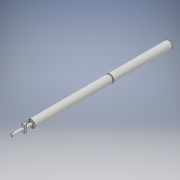
# Autodesk Inventor part: Lever
Saved by Autodesk Inventor 2018 (Build 220112000, 112)
## iProperties
Created: 2019-06-06
Part Number: Lever
Material: Generic
Document SubType Name: Modeling
Designer: aal_9
Density: 1 g/cm^3
Appearance: Default
Mass: 30.5385 g
Surface Area: 111.723 cm^2
Volume: 30.5385 cm^3
Author: aal_9
Autodesk Inventor part; units mm, degrees
ref_plane "YZ Plane" through (0, 0, 0) normal (1, 0, 0) x (0, 1, 0)
ref_plane "XZ Plane" through (0, 0, 0) normal (0, 1, 0) x (-1, 0, 0)
sketch "Sketch1" plane through (0, 0, 0) normal (0, 1, 0) x (-1, 0, 0)
  circle A0 centre (0, 0) radius 6
  dimension "d0" = 12
  constraints: 1 centre point, 1 coincident
  measures "d0" diameter of A0
extrude "Extrusion1" add sketch "Sketch1" along normal blind 250
sketch "Sketch2" plane through (0, 0, 0) normal (0, 0, 1) x (1, 0, 0)
  line L0 (-6, 0) -> (-6, 250) projected
  line L1 (-6, 155.5) -> (-4.875, 155.5)
  line L2 (-4.875, 155.5) -> (-4.875, 157)
  line L3 (-4.875, 157) -> (-6, 157)
  line L4 (-6, 157) -> (-6, 155.5)
  line L5 (0, 0) -> (0, 268.3776) construction
  line L6 (-6, 0) -> (6, 0) projected
  line L7 (6, 250) -> (-6, 250) projected
  dimension "d3" = 1.125
  dimension "d4" = 1.5
  dimension "d21" = 93
  constraints: 10 end point, 2 parallel, 1 horizontal, 1 perpendicular, 1 point on line, 1 vertical
  measures "d3" distance of L1.start L1.end
  measures "d4" distance of L1.end L2.end
  measures "d21" distance between parallel lines of L7 L3
revolve "Revolution1" cut sketch "Sketch2" angle 360 about axis through (0, 0, 0) along (0, 1, 0)
sketch "Sketch3" plane through (0, 0, 0) normal (0, 0, 1) x (1, 0, 0)
  circle A0 centre (0, 245) radius 2.5
  line L0 (6, 250) -> (-6, 250) projected
  point P0 (0, 0)
  dimension "d7" = 5
  dimension "d9" = 5
  constraints: 1 centre point
  measures "d7" diameter of A0
  measures "d9" distance from line of A0.centre L0
extrude "Extrusion2" cut sketch "Sketch3" along normal blind 2 and the other way blind 10
sketch "Sketch4" plane through (0, 250, 0) normal (0, 1, 0) x (1, 0, 0)
  point P0 (0, 0)
  point P1 (0, 0)
  constraints: 1 coincident
hole "Hole1" at (0, 250, 0) direction (0, -1, 0) diameter 2.459 depth 6 tip angle 118 thread size "M3x0.5" class "6H" standard "ANSI Metric M Profile"
sketch "Sketch5" plane through (0, 0, 0) normal (1, 0, 0) x (0, 1, 0)
  line L0 (250, -6) -> (250, 6) projected
  point P0 (0, 0)
  point P1 (220, 0)
  dimension "d22" = 30
  measures "d22" distance from line of L0 point (220, 0)
hole "Hole2" at (0, 220, 0) direction (-1, 0, 0) diameter 5 end through all
sketch "Sketch6" plane through (0, 0, 0) normal (0, -1, 0) x (1, 0, 0)
  circle A0 centre (0, 0) radius 2
  circle A1 centre (0, 0) radius 6
  dimension "d30" = 4
  dimension "d31" = 12
  constraints: 2 centre point, 2 coincident
  measures "d30" diameter of A0
  measures "d31" diameter of A1
extrude "Extrusion3" cut sketch "Sketch6" against normal blind 18.4
ref_plane "Work Plane1" through (0, 31.8, 0) normal (0, -1, 0) x (1, 0, 0)
sketch "Sketch7" plane through (0, 31.8, 0) normal (0, -1, 0) x (1, 0, 0)
  circle A0 centre (0, 0) radius 6
  circle A1 centre (0, 0) radius 2
  dimension "d35" = 12
  dimension "d36" = 4
  constraints: 2 centre point, 2 coincident
  measures "d35" diameter of A0
  measures "d36" diameter of A1
extrude "Extrusion4" cut sketch "Sketch7" along normal blind 9.4
sketch "Sketch9" plane through (0, 0, 0) normal (0, 0, 1) x (1, 0, 0)
  line L0 (2, 31.8) -> (2, 22.4) projected
  line L1 (6, 18.4) -> (-6, 18.4) projected
  line L2 (2, 22.4) -> (6, 22.4)
  line L3 (6, 22.4) -> (6, 18.4)
  line L4 (6, 18.4) -> (2, 18.4)
  line L5 (2, 18.4) -> (2, 22.4)
  line L6 (-2, 31.8) -> (-2, 22.4) projected
  line L7 (-6, 18.4) -> (-2, 18.4)
  line L8 (-2, 18.4) -> (-2, 22.4)
  line L9 (-2, 22.4) -> (-6, 22.4)
  line L10 (-6, 22.4) -> (-6, 18.4)
  point P0 (0, 0)
  dimension "d39" = 4
  constraints: 16 end point, 4 parallel, 3 point on line, 2 horizontal, 2 perpendicular
  measures "d39" distance of L8.end L9.end
extrude "Extrusion5" cut sketch "Sketch9" along normal through all both and the other way through all
sketch "Sketch10" plane through (0, 31.8, 0) normal (0, -1, 0) x (1, 0, 0)
  arc A0 (2.0552, 1.1503) -> (2.0552, -1.1503) centre (0, 0) ccw construction
  line L0 (0, 2.5) -> (0, -2.5) projected
  line L1 (2.0552, -6.3985) -> (2.6552, -6.3985)
  line L2 (2.6552, -6.3985) -> (2.6552, -2.1237)
  arc A1 (-2.0552, -2.7086) -> (2.0552, -2.7086) centre (0, 0) ccw
  arc A2 (2.6552, -2.1237) -> (2.6552, 2.1237) centre (0, 0) ccw
  line L3 (2.0552, -2.7086) -> (2.0552, -6.3985)
  line L4 (-2.0552, 7.8347) -> (-2.6552, 7.8347)
  line L5 (-2.6552, 7.8347) -> (-2.6552, 2.1237)
  line L6 (-2.0552, 2.7086) -> (-2.0552, 7.8347)
  arc A3 (2.6552, -2.1237) -> (-2.0552, 2.7086) centre (0, 0) ccw
  arc A4 (-2.6552, 2.1237) -> (2.0552, -2.7086) centre (0, 0) ccw
  arc A5 (2.0552, 2.7086) -> (-2.0552, 2.7086) centre (0, 0) ccw
  arc A6 (-2.6552, 2.1237) -> (-2.6552, -2.1237) centre (0, 0) ccw
  dimension "d59" = 0
  dimension "d60" = 0.6
  dimension "d62" = 0.6
  constraints: 16 point on circle, 12 end point, 7 centre point, 2 coincident, 2 parallel
  measures "d59" distance from line of A0.centre L0
  measures "d60" distance of L1.end L1.start
  measures "d62" distance of L4.end L4.start
extrude "Extrusion6" cut sketch "Sketch10" against normal blind 1
sketch "Sketch11" plane through (-2, 18.4, -5.6569) normal (-1, 0, 0) x (0, 0, 1)
  line L0 (3.6569, -18.4) -> (3.6569, 0) projected
  line L1 (7.6569, -18.4) -> (7.6569, 0) projected
  line L2 (3.6569, -18.4) -> (7.6569, -18.4)
  line L3 (7.6569, -18.4) -> (7.6569, -13.4)
  line L4 (7.6569, -13.4) -> (3.6569, -13.4)
  line L5 (3.6569, -13.4) -> (3.6569, -18.4)
  point P0 (5.6569, -18.4)
  dimension "d63" = 5
  constraints: 8 end point, 2 parallel, 2 point on line, 1 horizontal, 1 perpendicular
  measures "d63" distance between parallel lines of L4 L2
extrude "Extrusion7" cut sketch "Sketch11" against normal blind 0.5
body "Solid1"
